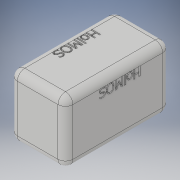
# Autodesk Inventor part: 7.3 Schienendteil
Saved by Autodesk Inventor 2018.3 (Build 223284000, 284)
## iProperties
Created: 2018-10-18
Part Number: 7.3 Schienendteil
Material: Generisch
Document SubType Name: Modeling
Designer: pgmadmin
Density: 1 g/cm^3
Appearance: Vorgabe
Author: pgmadmin
Autodesk Inventor part; units mm, degrees
ref_plane "YZ Plane" through (0, 0, 0) normal (1, 0, 0) x (0, 1, 0)
ref_plane "XZ Plane" through (0, 0, 0) normal (0, 1, 0) x (-1, 0, 0)
ref_plane "XY Plane" through (0, 0, 0) normal (0, 0, 1) x (1, 0, 0)
sketch "Skizze1" plane through (0, 0, 0) normal (0, 0, 1) x (1, 0, 0)
  line L0 (0, 0) -> (-22.3, 0)
  line L1 (-22.3, 0) -> (-22.3, 42)
  line L2 (-22.3, 42) -> (0, 42)
  line L3 (0, 42) -> (0, 0)
  line L4 (-19.3, 35) -> (-3, 35)
  line L5 (-3, 35) -> (-3, 33.4)
  line L6 (-3, 33.4) -> (-4.7, 33.4)
  line L7 (-4.7, 8.6) -> (-3, 8.6)
  line L8 (-3, 8.6) -> (-3, 7)
  line L9 (-3, 7) -> (-19.3, 7)
  line L10 (-19.3, 7) -> (-19.3, 35)
  line L11 (-4.7, 33.4) -> (-4.7, 8.6)
  line L12 (-11.15, 7) -> (-11.15, 0)
  line L13 (-11.15, 35) -> (-11.15, 42)
  dimension "d1" = 42
  dimension "d2" = 16.3
  dimension "d3" = 1.6
  dimension "d6" = 1.6
  dimension "d7" = 28
  dimension "d8" = 1.7
  dimension "d10" = 3
  dimension "d17" = 16.3
  dimension "d19" = 3
  constraints: 28 end point, 6 perpendicular, 4 midpoint, 2 horizontal, 2 parallel, 1 collinear, 1 vertical
  measures "d1" distance of L0.end L1.end
  measures "d2" distance of L4.start L4.end
  measures "d3" distance of L4.end L5.end
  measures "d6" distance of L7.end L8.end
  measures "d7" distance of L9.end L4.start
  measures "d8" distance of L6.end L5.end
  measures "d10" distance between parallel lines of L3 L5
  measures "d17" distance of L8.end L9.end
  measures "d19" distance between parallel lines of L1 L10
extrude "Extrusion1" add sketch "Skizze1" along normal blind 20 contours L0 L12 L9 L8 L7 L11 L6 L5 L4 L13 L2 L3 | L0 L1 L2 L13 L4 L10 L9 L12
sketch "Skizze2" plane through (0, 0, 20) normal (0, 0, 1) x (1, 0, 0)
  line L0 (0, 42) -> (-22.3, 42) projected
  line L1 (-22.3, 42) -> (0, 42)
  line L2 (0, 42) -> (0, 0)
  line L3 (0, 0) -> (-22.3, 0)
  line L4 (-22.3, 0) -> (-22.3, 42)
  constraints: 8 end point, 2 parallel, 1 horizontal, 1 perpendicular
extrude "Extrusion2" add sketch "Skizze2" along normal blind 5
fillet "Rundung1" radius 3 12 edges at (-11.15, 0, 0) (-22.3, 21, 0) (0, 21, 0) (-11.15, 42, 0) (0, 21, 25) (0, 0, 12.5) (-11.15, 0, 25) (-22.3, 0, 12.5) (-22.3, 21, 25) (-11.15, 42, 25) (0, 42, 12.5) (-22.3, 42, 12.5)
sketch "Skizze3" plane through (0, 0, 25) normal (0, 0, 1) x (1, 0, 0)
  line L0 (-19.3, 3) -> (-19.3, 39) projected
  line L1 (-19.3, 39) -> (-19.3, 3)
  line L2 (-19.3, 27.3865) -> (-19.3, 27.8517)
  line L3 (-19.3, 27.8517) -> (-17.5869, 27.8517)
  line L4 (-17.5869, 27.8517) -> (-17.5869, 29.4627)
  line L5 (-17.5869, 29.4627) -> (-19.3, 29.4627)
  line L6 (-19.3, 29.4627) -> (-19.3, 29.9279)
  line L7 (-19.3, 29.9279) -> (-15.8, 29.9279)
  line L8 (-15.8, 29.9279) -> (-15.8, 29.4627)
  line L9 (-15.8, 29.4627) -> (-17.1728, 29.4627)
  line L10 (-17.1728, 29.4627) -> (-17.1728, 27.8517)
  line L11 (-17.1728, 27.8517) -> (-15.8, 27.8517)
  line L12 (-15.8, 27.8517) -> (-15.8, 27.3865)
  line L13 (-15.8, 27.3865) -> (-19.3, 27.3865)
  spline S0 degree 2 poles (-17.9868, 24.5531) (-18.6505, 24.5531) (-19.3737, 25.1912) (-19.3737, 25.7245) knots 0 0 0 1 2 2 2
  spline S1 degree 2 poles (-19.3737, 25.7245) (-19.3737, 26.2719) (-18.6278, 26.8987) (-17.9868, 26.8987) knots 0 0 0 1 2 2 2
  spline S2 degree 2 poles (-17.9868, 26.8987) (-17.3288, 26.8987) (-16.5998, 26.252) (-16.5998, 25.7245) knots 0 0 0 1 2 2 2
  spline S3 degree 2 poles (-16.5998, 25.7245) (-16.5998, 25.1912) (-17.3259, 24.5531) (-17.9868, 24.5531) knots 0 0 0 1 2 2 2
  spline S4 degree 2 poles (-17.9868, 25.0097) (-17.4763, 25.0097) (-16.9799, 25.3813) (-16.9799, 25.7245) knots 0 0 0 1 2 2 2
  spline S5 degree 2 poles (-16.9799, 25.7245) (-16.9799, 26.0677) (-17.4763, 26.4421) (-17.9868, 26.4421) knots 0 0 0 1 2 2 2
  spline S6 degree 2 poles (-17.9868, 26.4421) (-18.4831, 26.4421) (-18.9937, 26.0677) (-18.9937, 25.7245) knots 0 0 0 1 2 2 2
  spline S7 degree 2 poles (-18.9937, 25.7245) (-18.9937, 25.3841) (-18.4917, 25.0097) (-17.9868, 25.0097) knots 0 0 0 1 2 2 2
  line L14 (-19.3, 23.6483) -> (-19.3, 24.0908)
  line L15 (-19.3, 24.0908) -> (-15.644, 24.0908)
  line L16 (-15.644, 24.0908) -> (-15.644, 23.6483)
  line L17 (-15.644, 23.6483) -> (-19.3, 23.6483)
  line L18 (-19.3, 19.9639) -> (-19.3, 20.4291)
  line L19 (-19.3, 20.4291) -> (-16.285, 20.4291)
  line L20 (-16.285, 20.4291) -> (-18.3357, 21.3424)
  line L21 (-18.3357, 21.3424) -> (-18.3357, 21.626)
  line L22 (-18.3357, 21.626) -> (-16.285, 22.5308)
  line L23 (-16.285, 22.5308) -> (-19.3, 22.5308)
  line L24 (-19.3, 22.5308) -> (-19.3, 22.9648)
  line L25 (-19.3, 22.9648) -> (-15.8, 22.9648)
  line L26 (-15.8, 22.9648) -> (-15.8, 22.3294)
  line L27 (-15.8, 22.3294) -> (-17.7485, 21.4558)
  line L28 (-17.7485, 21.4558) -> (-15.8, 20.6106)
  line L29 (-15.8, 20.6106) -> (-15.8, 19.9639)
  line L30 (-15.8, 19.9639) -> (-19.3, 19.9639)
  spline S8 degree 2 poles (-16.1999, 16.7788) (-16.4325, 16.5802) (-17.1132, 16.359) (-17.55, 16.359) knots 0 0 0 1 2 2 2
  spline S9 degree 2 poles (-17.55, 16.359) (-17.9754, 16.359) (-18.6647, 16.5746) (-18.8972, 16.7788) knots 0 0 0 1 2 2 2
  spline S10 degree 2 poles (-18.8972, 16.7788) (-19.1412, 16.9943) (-19.3737, 17.5644) (-19.3737, 17.9076) knots 0 0 0 1 2 2 2
  spline S11 degree 2 poles (-19.3737, 17.9076) (-19.3737, 18.2622) (-19.1327, 18.8294) (-18.8972, 19.0365) knots 0 0 0 1 2 2 2
  spline S12 degree 2 poles (-18.8972, 19.0365) (-18.6647, 19.2378) (-17.9811, 19.4534) (-17.55, 19.4534) knots 0 0 0 1 2 2 2
  spline S13 degree 2 poles (-17.55, 19.4534) (-17.1104, 19.4534) (-16.441, 19.235) (-16.1999, 19.0336) knots 0 0 0 1 2 2 2
  spline S14 degree 2 poles (-16.1999, 19.0336) (-15.9673, 18.8294) (-15.7263, 18.2593) (-15.7263, 17.9076) knots 0 0 0 1 2 2 2
  spline S15 degree 2 poles (-15.7263, 17.9076) (-15.7263, 17.5502) (-15.9759, 16.9773) (-16.1999, 16.7788) knots 0 0 0 1 2 2 2
  spline S16 degree 2 poles (-17.55, 16.844) (-17.204, 16.844) (-16.6679, 16.9943) (-16.4921, 17.1305) knots 0 0 0 1 2 2 2
  spline S17 degree 2 poles (-16.4921, 17.1305) (-16.3105, 17.2695) (-16.129, 17.6609) (-16.129, 17.9048) knots 0 0 0 1 2 2 2
  spline S18 degree 2 poles (-16.129, 17.9048) (-16.129, 18.1572) (-16.3049, 18.5373) (-16.4921, 18.6819) knots 0 0 0 1 2 2 2
  spline S19 degree 2 poles (-16.4921, 18.6819) (-16.6707, 18.8209) (-17.2096, 18.9684) (-17.55, 18.9684) knots 0 0 0 1 2 2 2
  spline S20 degree 2 poles (-17.55, 18.9684) (-18.2392, 18.9684) (-18.971, 18.3898) (-18.971, 17.9048) knots 0 0 0 1 2 2 2
  spline S21 degree 2 poles (-18.971, 17.9048) (-18.971, 17.4198) (-18.2392, 16.844) (-17.55, 16.844) knots 0 0 0 1 2 2 2
  spline S22 degree 2 poles (-19.3624, 14.8728) (-19.3624, 15.2528) (-19.2036, 15.7861) (-19.0901, 16.0215) knots 0 0 0 1 2 2 2
  line L31 (-19.0901, 16.0215) -> (-18.5058, 16.0215)
  line L32 (-18.5058, 16.0215) -> (-18.5058, 15.9874)
  spline S23 degree 2 poles (-18.5058, 15.9874) (-18.7214, 15.7577) (-18.9596, 15.1763) (-18.9596, 14.9068) knots 0 0 0 1 2 2 2
  spline S24 degree 2 poles (-18.9596, 14.9068) (-18.9596, 14.5211) (-18.6391, 14.1268) (-18.3754, 14.1268) knots 0 0 0 1 2 2 2
  spline S25 degree 2 poles (-18.3754, 14.1268) (-18.1655, 14.1268) (-17.9045, 14.3339) (-17.8393, 14.5579) knots 0 0 0 1 2 2 2
  spline S26 degree 2 poles (-17.8393, 14.5579) (-17.7939, 14.7196) (-17.7315, 14.9891) (-17.6805, 15.1904) knots 0 0 0 1 2 2 2
  spline S27 degree 2 poles (-17.6805, 15.1904) (-17.6323, 15.372) (-17.4876, 15.6584) (-17.3713, 15.769) knots 0 0 0 1 2 2 2
  spline S28 degree 2 poles (-17.3713, 15.769) (-17.255, 15.8768) (-16.943, 15.9959) (-16.7388, 15.9959) knots 0 0 0 1 2 2 2
  spline S29 degree 2 poles (-16.7388, 15.9959) (-16.3134, 15.9959) (-15.7376, 15.3323) (-15.7376, 14.8189) knots 0 0 0 1 2 2 2
  spline S30 degree 2 poles (-15.7376, 14.8189) (-15.7376, 14.5239) (-15.8539, 14.002) (-15.9645, 13.778) knots 0 0 0 1 2 2 2
  line L33 (-15.9645, 13.778) -> (-16.5204, 13.778)
  line L34 (-16.5204, 13.778) -> (-16.5204, 13.812)
  spline S31 degree 2 poles (-16.5204, 13.812) (-16.3673, 13.9793) (-16.1404, 14.5012) (-16.1404, 14.7877) knots 0 0 0 1 2 2 2
  spline S32 degree 2 poles (-16.1404, 14.7877) (-16.1404, 15.111) (-16.4438, 15.5109) (-16.6906, 15.5109) knots 0 0 0 1 2 2 2
  spline S33 degree 2 poles (-16.6906, 15.5109) (-16.9118, 15.5109) (-17.1756, 15.2755) (-17.2352, 15.0543) knots 0 0 0 1 2 2 2
  spline S34 degree 2 poles (-17.2352, 15.0543) (-17.2749, 14.9068) (-17.377, 14.4785) (-17.4195, 14.3367) knots 0 0 0 1 2 2 2
  spline S35 degree 2 poles (-17.4195, 14.3367) (-17.5301, 13.9765) (-17.9754, 13.6418) (-18.3016, 13.6418) knots 0 0 0 1 2 2 2
  spline S36 degree 2 poles (-18.3016, 13.6418) (-18.5087, 13.6418) (-18.9058, 13.8092) (-19.0447, 13.9595) knots 0 0 0 1 2 2 2
  spline S37 degree 2 poles (-19.0447, 13.9595) (-19.1979, 14.1268) (-19.3624, 14.5523) (-19.3624, 14.8728) knots 0 0 0 1 2 2 2
  point P0 (0, 0)
  constraints: 2 end point, 2 vertical
extrude "Extrusion3" cut sketch "Skizze3" against normal blind 2 contours L0 L3 L4 L5 L7 L8 L9 L10 L11 L12 L13 | S0 S1 L0 | L0 S1 S2 S3 S0 | L0 L15 L16 L17 | S22 L31 L32 S23 S24 S25 S26 S27 S28 S29 S30 L33 L34 S31 S32 S33 S34 S35 S36 S37 L0 | L0 S37 S22 | S11 S12 S13 S14 S15 S8 S9 S10 L0 | L0 S10 S11 | L0 L19 L20 L21 L22 L23 L25 L26 L27 L28 L29 L30
sketch "Skizze4" plane through (0, 3, 22) normal (1, 0, 0) x (0, 0, -1)
  line L0 (-3, 36) -> (0, 36) projected
  line L1 (0, 0) -> (-3, 0) projected
  line L2 (0, 36) -> (0, 0)
  line L3 (0, 24.3865) -> (0, 24.8517)
  line L4 (0, 24.8517) -> (1.7131, 24.8517)
  line L5 (1.7131, 24.8517) -> (1.7131, 26.4627)
  line L6 (1.7131, 26.4627) -> (0, 26.4627)
  line L7 (0, 26.4627) -> (0, 26.9279)
  line L8 (0, 26.9279) -> (3.5, 26.9279)
  line L9 (3.5, 26.9279) -> (3.5, 26.4627)
  line L10 (3.5, 26.4627) -> (2.1272, 26.4627)
  line L11 (2.1272, 26.4627) -> (2.1272, 24.8517)
  line L12 (2.1272, 24.8517) -> (3.5, 24.8517)
  line L13 (3.5, 24.8517) -> (3.5, 24.3865)
  line L14 (3.5, 24.3865) -> (0, 24.3865)
  spline S0 degree 2 poles (1.3132, 21.5531) (0.6495, 21.5531) (-0.0737, 22.1912) (-0.0737, 22.7245) knots 0 0 0 1 2 2 2
  spline S1 degree 2 poles (-0.0737, 22.7245) (-0.0737, 23.2719) (0.6722, 23.8987) (1.3132, 23.8987) knots 0 0 0 1 2 2 2
  spline S2 degree 2 poles (1.3132, 23.8987) (1.9712, 23.8987) (2.7002, 23.252) (2.7002, 22.7245) knots 0 0 0 1 2 2 2
  spline S3 degree 2 poles (2.7002, 22.7245) (2.7002, 22.1912) (1.9741, 21.5531) (1.3132, 21.5531) knots 0 0 0 1 2 2 2
  spline S4 degree 2 poles (1.3132, 22.0097) (1.8237, 22.0097) (2.3201, 22.3813) (2.3201, 22.7245) knots 0 0 0 1 2 2 2
  spline S5 degree 2 poles (2.3201, 22.7245) (2.3201, 23.0677) (1.8237, 23.4421) (1.3132, 23.4421) knots 0 0 0 1 2 2 2
  spline S6 degree 2 poles (1.3132, 23.4421) (0.8169, 23.4421) (0.3063, 23.0677) (0.3063, 22.7245) knots 0 0 0 1 2 2 2
  spline S7 degree 2 poles (0.3063, 22.7245) (0.3063, 22.3841) (0.8083, 22.0097) (1.3132, 22.0097) knots 0 0 0 1 2 2 2
  line L15 (0, 20.6483) -> (0, 21.0908)
  line L16 (0, 21.0908) -> (3.656, 21.0908)
  line L17 (3.656, 21.0908) -> (3.656, 20.6483)
  line L18 (3.656, 20.6483) -> (0, 20.6483)
  line L19 (0, 16.9639) -> (0, 17.4291)
  line L20 (0, 17.4291) -> (3.015, 17.4291)
  line L21 (3.015, 17.4291) -> (0.9643, 18.3424)
  line L22 (0.9643, 18.3424) -> (0.9643, 18.626)
  line L23 (0.9643, 18.626) -> (3.015, 19.5308)
  line L24 (3.015, 19.5308) -> (0, 19.5308)
  line L25 (0, 19.5308) -> (0, 19.9648)
  line L26 (0, 19.9648) -> (3.5, 19.9648)
  line L27 (3.5, 19.9648) -> (3.5, 19.3294)
  line L28 (3.5, 19.3294) -> (1.5515, 18.4558)
  line L29 (1.5515, 18.4558) -> (3.5, 17.6106)
  line L30 (3.5, 17.6106) -> (3.5, 16.9639)
  line L31 (3.5, 16.9639) -> (0, 16.9639)
  spline S8 degree 2 poles (3.1001, 13.7788) (2.8675, 13.5802) (2.1868, 13.359) (1.75, 13.359) knots 0 0 0 1 2 2 2
  spline S9 degree 2 poles (1.75, 13.359) (1.3246, 13.359) (0.6353, 13.5746) (0.4028, 13.7788) knots 0 0 0 1 2 2 2
  spline S10 degree 2 poles (0.4028, 13.7788) (0.1588, 13.9943) (-0.0737, 14.5644) (-0.0737, 14.9076) knots 0 0 0 1 2 2 2
  spline S11 degree 2 poles (-0.0737, 14.9076) (-0.0737, 15.2622) (0.1673, 15.8294) (0.4028, 16.0365) knots 0 0 0 1 2 2 2
  spline S12 degree 2 poles (0.4028, 16.0365) (0.6353, 16.2378) (1.3189, 16.4534) (1.75, 16.4534) knots 0 0 0 1 2 2 2
  spline S13 degree 2 poles (1.75, 16.4534) (2.1896, 16.4534) (2.859, 16.235) (3.1001, 16.0336) knots 0 0 0 1 2 2 2
  spline S14 degree 2 poles (3.1001, 16.0336) (3.3327, 15.8294) (3.5737, 15.2593) (3.5737, 14.9076) knots 0 0 0 1 2 2 2
  spline S15 degree 2 poles (3.5737, 14.9076) (3.5737, 14.5502) (3.3241, 13.9773) (3.1001, 13.7788) knots 0 0 0 1 2 2 2
  spline S16 degree 2 poles (1.75, 13.844) (2.096, 13.844) (2.6321, 13.9943) (2.8079, 14.1305) knots 0 0 0 1 2 2 2
  spline S17 degree 2 poles (2.8079, 14.1305) (2.9895, 14.2695) (3.171, 14.6609) (3.171, 14.9048) knots 0 0 0 1 2 2 2
  spline S18 degree 2 poles (3.171, 14.9048) (3.171, 15.1572) (2.9951, 15.5373) (2.8079, 15.6819) knots 0 0 0 1 2 2 2
  spline S19 degree 2 poles (2.8079, 15.6819) (2.6293, 15.8209) (2.0904, 15.9684) (1.75, 15.9684) knots 0 0 0 1 2 2 2
  spline S20 degree 2 poles (1.75, 15.9684) (1.0608, 15.9684) (0.329, 15.3898) (0.329, 14.9048) knots 0 0 0 1 2 2 2
  spline S21 degree 2 poles (0.329, 14.9048) (0.329, 14.4198) (1.0608, 13.844) (1.75, 13.844) knots 0 0 0 1 2 2 2
  spline S22 degree 2 poles (-0.0624, 11.8728) (-0.0624, 12.2528) (0.0964, 12.7861) (0.2099, 13.0215) knots 0 0 0 1 2 2 2
  line L32 (0.2099, 13.0215) -> (0.7942, 13.0215)
  line L33 (0.7942, 13.0215) -> (0.7942, 12.9874)
  spline S23 degree 2 poles (0.7942, 12.9874) (0.5786, 12.7577) (0.3404, 12.1763) (0.3404, 11.9068) knots 0 0 0 1 2 2 2
  spline S24 degree 2 poles (0.3404, 11.9068) (0.3404, 11.5211) (0.6609, 11.1268) (0.9246, 11.1268) knots 0 0 0 1 2 2 2
  spline S25 degree 2 poles (0.9246, 11.1268) (1.1345, 11.1268) (1.3955, 11.3339) (1.4607, 11.5579) knots 0 0 0 1 2 2 2
  spline S26 degree 2 poles (1.4607, 11.5579) (1.5061, 11.7196) (1.5685, 11.9891) (1.6195, 12.1904) knots 0 0 0 1 2 2 2
  spline S27 degree 2 poles (1.6195, 12.1904) (1.6677, 12.372) (1.8124, 12.6584) (1.9287, 12.769) knots 0 0 0 1 2 2 2
  spline S28 degree 2 poles (1.9287, 12.769) (2.045, 12.8768) (2.357, 12.9959) (2.5612, 12.9959) knots 0 0 0 1 2 2 2
  spline S29 degree 2 poles (2.5612, 12.9959) (2.9866, 12.9959) (3.5624, 12.3323) (3.5624, 11.8189) knots 0 0 0 1 2 2 2
  spline S30 degree 2 poles (3.5624, 11.8189) (3.5624, 11.5239) (3.4461, 11.002) (3.3355, 10.778) knots 0 0 0 1 2 2 2
  line L34 (3.3355, 10.778) -> (2.7796, 10.778)
  line L35 (2.7796, 10.778) -> (2.7796, 10.812)
  spline S31 degree 2 poles (2.7796, 10.812) (2.9327, 10.9793) (3.1596, 11.5012) (3.1596, 11.7877) knots 0 0 0 1 2 2 2
  spline S32 degree 2 poles (3.1596, 11.7877) (3.1596, 12.111) (2.8562, 12.5109) (2.6094, 12.5109) knots 0 0 0 1 2 2 2
  spline S33 degree 2 poles (2.6094, 12.5109) (2.3882, 12.5109) (2.1244, 12.2755) (2.0648, 12.0543) knots 0 0 0 1 2 2 2
  spline S34 degree 2 poles (2.0648, 12.0543) (2.0251, 11.9068) (1.923, 11.4785) (1.8805, 11.3367) knots 0 0 0 1 2 2 2
  spline S35 degree 2 poles (1.8805, 11.3367) (1.7699, 10.9765) (1.3246, 10.6418) (0.9984, 10.6418) knots 0 0 0 1 2 2 2
  spline S36 degree 2 poles (0.9984, 10.6418) (0.7913, 10.6418) (0.3942, 10.8092) (0.2553, 10.9595) knots 0 0 0 1 2 2 2
  spline S37 degree 2 poles (0.2553, 10.9595) (0.1021, 11.1268) (-0.0624, 11.5523) (-0.0624, 11.8728) knots 0 0 0 1 2 2 2
  point P0 (22, -3)
  constraints: 2 end point, 2 vertical
extrude "Extrusion4" cut sketch "Skizze4" against normal blind 2 contours L8 L9 L10 L11 L12 L13 L14 L2 L4 L5 L6 | S22 L32 L33 S23 S24 S25 S26 S27 S28 S29 S30 L34 L35 S31 S32 S33 S34 S35 S36 S37 L2 | L2 S37 S22 | S11 S12 S13 S14 S15 S8 S9 S10 L2 | L2 S10 S11 | L26 L27 L28 L29 L30 L31 L2 L20 L21 L22 L23 L24 | L16 L17 L18 L2 | S1 S2 S3 S0 L2 | L2 S0 S1
